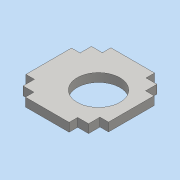
# Autodesk Inventor part: Camera-Holder_Bearing-Ring-Middle-Left
Saved by Autodesk Inventor 2016 SP1 (Build 200210100, 210)
## iProperties
Created: 2016-01-20
Part Number: Camera-Holder_Bearing-Ring-Middle-Left
Material: Generic
Document SubType Name: Modeling
Designer: Mohamed A.
Density: 1 g/cm^3
Appearance: Default
Author: Mohamed A.
Autodesk Inventor part; units mm, degrees
ref_plane "YZ Plane" through (0, 0, 0) normal (1, 0, 0) x (0, 1, 0)
ref_plane "XZ Plane" through (0, 0, 0) normal (0, 1, 0) x (-1, 0, 0)
ref_plane "XY Plane" through (0, 0, 0) normal (0, 0, 1) x (1, 0, 0)
sketch "Sketch1" plane through (0, 0, 0) normal (0, 0, 1) x (1, 0, 0)
  circle A0 centre (0, 0) radius 7.5
  line L0 (11.4997, 8) -> (8.4997, 8)
  line L1 (8.4997, 8) -> (8.4997, 12)
  line L2 (8.4997, -12) -> (8.4997, -8)
  line L3 (8.4997, -8) -> (11.4997, -8)
  line L4 (-10.667, -15) -> (-10.667, -12)
  line L5 (-10.667, -12) -> (-14.5003, -12)
  line L6 (4.6663, -15) -> (4.6663, -12)
  line L7 (4.6663, -12) -> (8.4997, -12)
  line L8 (-17.5003, -8) -> (-14.5003, -8)
  line L9 (-14.5003, -8) -> (-14.5003, -12)
  line L10 (-17.5003, 8) -> (-14.5003, 8)
  line L11 (-14.5003, 8) -> (-14.5003, 12)
  line L12 (-10.667, 15) -> (-10.667, 12)
  line L13 (-10.667, 12) -> (-14.5003, 12)
  line L14 (8.4997, 12) -> (4.6663, 12)
  line L15 (4.6663, 12) -> (4.6663, 15)
  line L16 (11.4997, 8) -> (11.4997, -8)
  line L17 (-10.667, 15) -> (4.6663, 15)
  line L18 (-17.5003, -8) -> (-17.5003, 8)
  line L19 (4.6663, -15) -> (-10.667, -15)
  line L20 (11.4997, -7) -> (11.4997, 8)
  line L21 (-20.9424, 0) -> (31.3224, 0) construction
  line L22 (-0.0003, 36) -> (-0.0003, -23) construction
  dimension "d0" = 15
  dimension "d3" = 3
  dimension "d5" = 3
  dimension "d6" = 3
  dimension "d15" = 30
  dimension "d16" = 3
  dimension "d22" = 8.5
  dimension "d23" = 14.5
  dimension "d24" = 23
  dimension "d25" = 15.3333
  dimension "d26" = 24
  dimension "d27" = 16
  constraints: 46 end point, 12 point on line, 8 perpendicular, 4 horizontal, 3 collinear, 2 parallel, 2 vertical, 1 centre point, 1 coincident, 1 other
  measures "d0" diameter of A0
  measures "d3" distance of L0.start L0.end
  measures "d5" distance of L8.start L8.end
  measures "d6" distance of L12.start L12.end
  measures "d15" distance between parallel lines of L19 L17
  measures "d16" distance of L6.start L6.end
  measures "d22" distance between parallel lines of L1 L22
  measures "d23" distance between parallel lines of L22 L11
  measures "d24" distance between parallel lines of L11 L1
  measures "d25" distance between parallel lines of L12 L15
  measures "d26" distance between parallel lines of L7 L14
  measures "d27" distance between parallel lines of L3 L0
extrude "Extrusion1" add sketch "Sketch1" along normal mid plane 3
equation "\"d25\" = 0.666667 * d24"
equation "\"d27\" = 0.666667 * d26"
body "Solid1"
